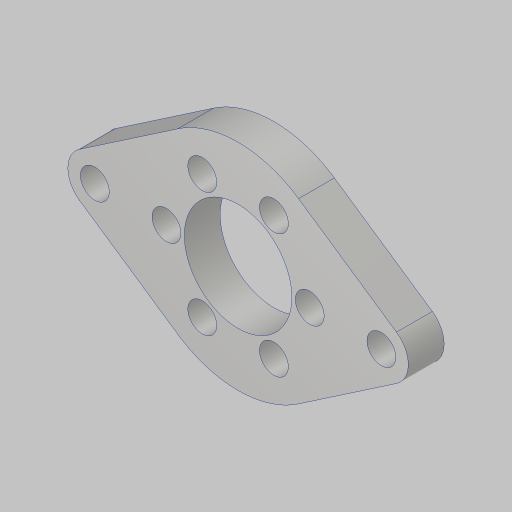
# Autodesk Inventor part: GP6-005
Saved by Autodesk Inventor 2023.5 (Build 275446000, 446)
## iProperties
Created: 2025-02-23
Part Number: GP6-005
Material: Aluminum 6061
Document SubType Name: Modeling
Designer: slick
Density: 2.7 g/cm^3
Appearance: Aluminum - Flat
Author: slick
Autodesk Inventor part; units mm, degrees
ref_plane "YZ Plane" through (0, 0, 0) normal (1, 0, 0) x (0, 1, 0)
ref_plane "XZ Plane" through (0, 0, 0) normal (0, 1, 0) x (-1, 0, 0)
ref_plane "XY Plane" through (0, 0, 0) normal (0, 0, 1) x (1, 0, 0)
sketch "Sketch1" plane through (0, 0, 0) normal (0, 0, 1) x (1, 0, 0)
  circle A0 centre (-25.4, 0) radius 4.7625 construction
  circle A1 centre (25.4, 0) radius 4.7625 construction
  line L0 (-25.4, 0) -> (25.4, 0) construction
  circle A2 centre (0, 0) radius 19.05 construction
  line L1 (-28.0789, 3.9376) -> (-10.7156, 15.7505)
  line L2 (10.7156, 15.7505) -> (28.0789, 3.9376)
  line L3 (28.0789, -3.9376) -> (10.7156, -15.7505)
  line L4 (-10.7156, -15.7505) -> (-28.0789, -3.9376)
  arc A3 (-28.0789, 3.9376) -> (-28.0789, -3.9376) centre (-25.4, 0) ccw
  arc A4 (28.0789, -3.9376) -> (28.0789, 3.9376) centre (25.4, 0) ccw
  arc A5 (10.7156, 15.7505) -> (-10.7156, 15.7505) centre (0, 0) ccw
  arc A6 (-10.7156, -15.7505) -> (10.7156, -15.7505) centre (0, 0) ccw
  circle A7 centre (0, 0) radius 9.525
  circle A8 centre (0, 0) radius 12.7 construction
  line L5 (0, 0) -> (-12.7, 0) construction
  point P0 (6.35, 10.9985)
  point P1 (-6.35, 10.9985)
  point P2 (-6.35, -10.9985)
  point P3 (6.35, -10.9985)
  point P4 (12.7, 0)
  dimension "d5" = 25.4
  dimension "d0" = 9.525
  dimension "d1" = 9.525
  dimension "d2" = 50.8
  dimension "d3" = 38.1
  dimension "d4" = 19.05
  dimension "d8" = 360
  constraints: 16 point on circle, 12 end point, 8 centre point, 8 coincident, 8 tangent, 1 collinear, 1 horizontal, 1 midpoint, 10 other
  measures "d0" diameter of A0
  measures "d1" diameter of A1
  measures "d2" distance of L0.start L0.end
  measures "d3" diameter of A2
  measures "d4" diameter of A7
extrude "Extrusion1" add sketch "Sketch1" along normal blind 6.35
hole "Hole1" at (6.35, 10.9985, 0) at (-6.35, 10.9985, 0) at (-12.7, 0, 0) at (-6.35, -10.9985, 0) at (6.35, -10.9985, 0) at (25.4, 0, 0) at (-25.4, 0, 0) at (12.7, 0, 0) direction (0, 0, 1) diameter 5.1054 end through all clearance for "Flat Head Machine Screw (82)" size "#10" standard "Ansi Unified Screw Threads"
body "Solid1"
